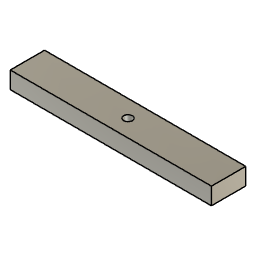
Soporte cámaras global (Autodesk Fusion 360 design; units mm, degrees)
Autodesk Fusion 360 part; units mm, degrees
sketch "Boceto1" plane through (0, 0, 0) normal (0, 0, 1) x (1, 0, 0)
  line L0 (65.1, -11.1) -> (-65.1, -11.1)
  line L1 (-65.1, -11.1) -> (-65.1, 11.1)
  line L2 (-65.1, 11.1) -> (65.1, 11.1)
  line L3 (65.1, 11.1) -> (65.1, -11.1)
  line L4 (65.1, -11.1) -> (-65.1, 11.1) construction
  line L5 (-65.1, -11.1) -> (65.1, 11.1) construction
  line L6 (0, 11.1) -> (0, -11.1) construction
  line L7 (-65.1, 0) -> (65.1, 0) construction
  circle A0 centre (20.4, 0) radius 5.55
  circle A1 centre (20.4, 0) radius 1.175
  circle A2 centre (-20.4, 0) radius 5.55
  circle A3 centre (-20.4, 0) radius 1.175
  circle A4 centre (31.5, 0) radius 5.55
  circle A5 centre (31.5, 0) radius 1.175
  circle A6 centre (-31.5, 0) radius 5.55
  circle A7 centre (-31.5, 0) radius 1.175
  circle A8 centre (42.6, 0) radius 5.55
  circle A9 centre (42.6, 0) radius 1.175
  circle A10 centre (-42.6, 0) radius 1.175
  circle A11 centre (-42.6, 0) radius 5.55
  dimension "d9" = 22.2
  dimension "d14" = 11.1
  dimension "d15" = 2.35
  dimension "d16" = 20.4
  dimension "d17" = 11.1
  dimension "d18" = 2.35
  dimension "d19" = 31.5
  dimension "d20" = 11.1
  dimension "d21" = 2.35
  dimension "d22" = 42.6
  dimension "d23" = 22.5
  constraint horizontal L0
  constraint perpendicular L0 L1
  constraint parallel L0 L2
  constraint parallel L1 L3
  constraint coincident L4 origin
  constraint coincident L5 origin
  constraint midpoint L2 L6.start
  constraint midpoint L0 L6.end
  constraint midpoint L1 L7.start
  constraint midpoint L3 L7.end
  constraint coincident L7 A0.centre
  constraint concentric A0 A1
  constraint symmetric L6 A0 A2
  constraint symmetric L6 A1 A3
  constraint coincident L7 A4.centre
  constraint concentric A4 A5
  constraint symmetric L6 A4 A6
  constraint symmetric L6 A5 A7
  constraint coincident L7 A8.centre
  constraint concentric A8 A9
  constraint symmetric L6 A8 A11
  constraint symmetric L6 A9 A10
  measures "d9" distance of L0.end L1.end
  measures "d14" diameter of A0
  measures "d15" diameter of A1
  measures "d16" distance of origin A0.centre
  measures "d17" diameter of A4
  measures "d18" diameter of A5
  measures "d19" distance of origin A4.centre
  measures "d20" diameter of A8
  measures "d21" diameter of A9
  measures "d22" distance of origin A8.centre
  measures "d23" distance of L7.end A8.centre
extrude "Extruir1" add sketch "Boceto1" along normal blind 11 contours L0 L1 L2 L3 | A0 | A8 | A4 | A1 | A2 | A11 | A6 | A3 | A5 | A7 | A9 | A10
extrude "Extruir2" cut sketch "Boceto1" along normal blind 2.45 contours A0 | A8 | A4 | A2 | A11 | A6
extrude "Extruir3" cut sketch "Boceto1" along normal blind 4.9 contours A1 | A3 | A5 | A7 | A9 | A10
sketch "Boceto2" plane through (0, 0, 11) normal (0, 0, 1) x (-1, 0, 0)
  line L0 (-65.1, -11.1) -> (65.1, -11.1)
  line L1 (65.1, -11.1) -> (65.1, 11.1)
  line L2 (65.1, 11.1) -> (-65.1, 11.1)
  line L3 (-65.1, 11.1) -> (-65.1, -11.1)
  line L4 (65.1, 0) -> (-65.1, 0) construction
  line L5 (0, 11.1) -> (0, -11.1) construction
  circle A0 centre (0, 0) radius 2.8
  dimension "d31" = 5.6
  constraint midpoint L1 L4.start
  constraint midpoint L3 L4.end
  constraint midpoint L2 L5.start
  constraint midpoint L0 L5.end
  constraint coincident L5 A0.centre
  constraint coincident L4 A0.centre
  measures "d31" diameter of A0
extrude "Extruir4" cut sketch "Boceto2" against normal blind 6 contours A0
equation "grosor1 = 2.8 mm"
equation "grosor2 = 2 mm"
equation "grosor3 = 7.5 mm"
equation "tolerancia = 0.1 mm"
equation "diametro_grande_iman = 11 mm"
equation "diametro_pequeno_iman = 2.25 mm"
equation "altura_grande_iman = 2.45 mm"
equation "altura_pequena_iman = 2.45 mm"
equation "d9 = 18 mm + tolerancia * 2 + grosor2 * 2"
equation "DIP_pequena = 41 mm"
equation "DIP_media = 63 mm"
equation "d14 = diametro_grande_iman + tolerancia"
equation "d15 = diametro_pequeno_iman + tolerancia"
equation "d16 = ( DIP_media - ( ( diametro_grande_iman + tolerancia ) * 2 ) ) / 2"
equation "d17 = diametro_grande_iman + tolerancia"
equation "d18 = diametro_pequeno_iman + tolerancia"
equation "d19 = DIP_media / 2"
equation "d20 = diametro_grande_iman + tolerancia"
equation "d21 = diametro_pequeno_iman + tolerancia"
equation "d22 = ( DIP_media + ( ( diametro_grande_iman + tolerancia ) * 2 ) ) / 2"
equation "grosor4 = 11 mm"
equation "d27 = altura_grande_iman"
equation "d29 = altura_pequena_iman + altura_grande_iman"
equation "d31 = 5.5 mm + tolerancia"
